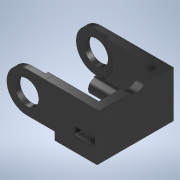
# Autodesk Inventor part: shroud left half
Saved by Autodesk Inventor 2020.4 (Build 244396000, 396)
## iProperties
Created: 2021-02-25
Part Number: shroud left half
Material: ABS Plastic
Document SubType Name: Modeling
Designer: AOB
Mass: 4.98213 g
Surface Area: 42.0816 cm^2
Volume: 4.70012 cm^3
Density: 1.06 g/cm^3
Appearance: Glossy - Black
Author: AOB
Autodesk Inventor part; units mm, degrees
ref_plane "YZ Plane" through (0, 0, 0) normal (1, 0, 0) x (0, 1, 0)
ref_plane "XZ Plane" through (0, 0, 0) normal (0, 1, 0) x (-1, 0, 0)
sketch "Sketch1" plane through (0, 0, 0) normal (0, 0, 1) x (1, 0, 0)
  line L0 (27, 0.0394) -> (27, 4.6148)
  line L1 (27.0072, 7.5) -> (27, 4.6148)
  arc A0 (26, -10.4606) -> (27, -9.4606) centre (26, -9.4606) ccw
  line L2 (27.0072, 7.5) -> (7.0216, 7.5)
  line L3 (7.0224, 7.5) -> (13.0399, 7.5)
  line L4 (7.0224, 7.5) -> (7.7962, 7.5)
  arc A1 (0, 7.5) -> (0.0224, -7.5) centre (0, 0) ccw
  line L5 (7.0224, 7.5) -> (0, 7.5)
  line L6 (0.0224, -7.5) -> (10.5224, -7.5)
  line L7 (26, -10.4606) -> (10.5224, -10.4606)
  line L8 (10.5224, -10.4606) -> (10.5224, -7.5)
  line L9 (25, -5.0606) -> (20.5, -5.0606)
  line L10 (25.5, -2.1068) -> (18, -2.1068)
  line L11 (18, -2.1068) -> (18, -4.5606)
  line L12 (18.5, -5.0606) -> (20.5, -5.0606)
  line L13 (18, -4.5606) -> (18.5, -5.0606)
  line L14 (27, 0.0394) -> (27, -9.4606)
  line L15 (27, -5.4606) -> (27, -9.4606)
  line L16 (25.5, -2.1068) -> (25.5, -4.5606)
  line L17 (25, -5.0606) -> (25.5, -4.5606)
  point P0 (27, -6.5436)
  point P1 (25.5, -5.0606)
  dimension "d3" = 1
  dimension "d66" = 10.5
  dimension "d77" = 5.4
  constraints: 36 end point, 6 point on line, 5 horizontal, 4 point on circle, 3 perpendicular, 3 tangent, 2 centre point, 2 vertical, 1 coincident
  measures "d3" radius of A0
  measures "d66" distance from line of L6.start L8
  measures "d77" distance between parallel lines of L7 L9
extrude "Extrusion1" add sketch "Sketch1" along normal blind 3
sketch "Sketch3" plane through (0, 0, 0) normal (0, 0, -1) x (-1, 0, 0)
  line L0 (-20.0398, -7.5) -> (-10.4968, -7.5)
  line L1 (-14.6929, -10.4606) -> (-26, -10.4606)
  line L2 (-27, -9.4606) -> (-27, -9.4606)
  line L3 (-14.6929, -10.4606) -> (-10.4968, -10.4606)
  line L4 (-10.4968, -7.5) -> (-10.4968, -7.5)
  line L5 (-10.4968, -7.5) -> (-10.4968, -10.4606)
  line L6 (-27, -9.4606) -> (-27, 4.6148) projected
  line L7 (-27, 4.6148) -> (-27.0072, 7.5) projected
  line L8 (-10.5224, -10.4606) -> (-26, -10.4606) projected
  arc A0 (-27, -9.4606) -> (-26, -10.4606) centre (-26, -9.4606) ccw projected
  line L9 (-27.0072, 7.5) -> (-24.0072, 7.5)
  line L10 (-18, -2.1068) -> (-25.5, -2.1068) projected
  line L11 (-25.5, -2.1068) -> (-25.5, -4.5606) projected
  line L12 (-25.5, -4.5606) -> (-25, -5.0606) projected
  line L13 (-25, -5.0606) -> (-18.5, -5.0606) projected
  line L14 (-24.0072, 7.5) -> (-24.0072, -2.1068)
  line L15 (-18, -2.1068) -> (-25.5, -2.1068) projected
  line L16 (-25, -5.0606) -> (-18.5, -5.0606) projected
  line L17 (-24.0072, -5.0606) -> (-24.0072, -7.5)
  line L18 (-24.0072, -7.5) -> (-20.0398, -7.5)
  point P0 (-24.0072, -2.1068)
  dimension "d84" = 3
  constraints: 20 end point, 4 point on line, 3 perpendicular, 1 vertical
  measures "d84" distance of L7.end L9.end
extrude "Extrusion3" add sketch "Sketch3" along normal blind 11
ref_plane "Work Plane1" through (0, 0, -11) normal (0, 0, -1) x (-1, 0, 0)
sketch "Sketch4" plane through (24.0072, 6.9501, 0) normal (-1, 0, 0) x (0, 0, 1)
  circle A0 centre (-11, -6) radius 2.5
  point P0 (0, -6.9501)
  dimension "d22" = 5
  constraints: 1 centre point
  measures "d22" diameter of A0
extrude "Extrusion4" add sketch "Sketch4" along normal blind 12.5
sketch "Sketch6" plane through (0, 0, 0) normal (0, 0, -1) x (-1, 0, 0)
  arc A0 (-5.0224, 5.57) -> (0, 7.5) centre (0, 0) ccw
  arc A1 (5.0224, 5.5902) -> (0, 7.5) centre (0, -0.0589) ccw
  line L0 (-5.0224, 5.57) -> (-5.0224, 7.5)
  line L1 (-5.0224, 7.5) -> (-5.0224, 5.57)
  line L2 (-7.0216, 7.5) -> (0, 7.5)
  line L3 (-5.0224, 7.5) -> (0, 7.5)
  circle A2 centre (0, -0.0589) radius 4.5
  point P0 (5.0224, 5.5902)
  dimension "d37" = 9
  constraints: 8 end point, 4 point on circle, 3 centre point, 2 coincident, 2 collinear, 1 tangent, 1 vertical
  measures "d37" diameter of A2
extrude "Extrusion8" cut sketch "Sketch6" along normal mid plane 2 contours L0 L2 A0 | A2
extrude "Extrusion9" cut sketch "Sketch6" against normal through all contours A2
mirror "Mirror4" about plane through (0, 0, -11) normal (0, 0, -1) of "Extrusion1", "Extrusion3", "Extrusion8", "Extrusion9"
sketch "Sketch8" plane through (24.0072, 6.9501, 0) normal (-1, 0, 0) x (0, 0, 1)
  line L0 (-10.9969, -2.5) -> (-10.9969, 3.2869)
  circle A0 centre (-10.9969, 3.2869) radius 4.0015
  line L1 (-10.9969, 1) -> (-10.9969, 3.2869)
  circle A1 centre (-11, -6) radius 2.5 projected
  dimension "d52" = 5.7869
  dimension "d53" = 8.003
  dimension "d85" = 3.5
  constraints: 4 end point, 2 vertical, 1 centre point, 1 coincident, 1 collinear
  measures "d52" distance of L0.end L0.start
  measures "d53" diameter of A0
  measures "d85" distance of A1.centre L0.start
extrude "Extrusion11" cut sketch "Sketch8" against normal blind 10 contours A0
body "Solid1"
